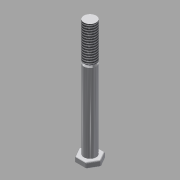
# Autodesk Inventor part: CIM Mount Bolt
Saved by Autodesk Inventor 2013 (Build 170138000, 138)
## iProperties
Created: 2013-01-18
Part Number: CIM Mount Bolt
Material: Aluminum 6061-AHC
Document SubType Name: Modeling
Designer: Naphat
Density: 1 g/cm^3
Author: Naphat
Autodesk Inventor part; units mm, degrees
ref_plane "YZ Plane" through (0, 0, 0) normal (1, 0, 0) x (0, 1, 0)
ref_plane "XZ Plane" through (0, 0, 0) normal (0, 1, 0) x (-1, 0, 0)
ref_plane "XY Plane" through (0, 0, 0) normal (0, 0, 1) x (1, 0, 0)
sketch "Sketch1" plane through (0, 0, 0) normal (0, 1, 0) x (-1, 0, 0)
  circle A0 centre (0, 0) radius 5
  dimension "d0" = 10
  constraints: 1 centre point, 1 coincident
  measures "d0" diameter of A0
extrude "Extrusion1" add sketch "Sketch1" along normal blind 65
sketch "Sketch2" plane through (0, 65, 0) normal (0, 1, 0) x (1, 0, 0)
  circle A0 centre (0, 0) radius 5 projected
  dimension "d38" = 10
  measures "d38" diameter of A0
chamfer "Chamfer1" distance 1 angle 45 1 edges at (5, 65, 0)
extrude "Extrusion2" add sketch "Sketch2" along normal blind 30
chamfer "Chamfer2" distance 1 angle 45 1 edges at (-5, 65, 0)
sketch "Sketch3" plane through (0, 0, 0) normal (0, -1, 0) x (1, 0, 0)
  line L0 (0, 0) -> (0, 0) construction
  line L1 (4.5, -7.7942) -> (-4.5, -7.7942)
  line L2 (-4.5, -7.7942) -> (-9, 0)
  line L3 (-9, 0) -> (-4.5, 7.7942)
  line L4 (-4.5, 7.7942) -> (4.5, 7.7942)
  line L5 (4.5, 7.7942) -> (9, 0)
  line L6 (9, 0) -> (4.5, -7.7942)
  circle A0 centre (0, 0) radius 5 projected
  line L7 (-4.5, -7.7942) -> (4.5, 7.7942) construction
  line L8 (-4.5, 7.7942) -> (4.5, -7.7942) construction
  dimension "d21" = 9
  dimension "d22" = 9
  dimension "d23" = 120
  dimension "d24" = 9
  dimension "d25" = 9
  dimension "d26" = 120
  dimension "d34" = 9
  dimension "d36" = 0
  dimension "d37" = 0
  constraints: 18 end point, 3 parallel, 1 perpendicular
  measures "d21" distance of L1.start L1.end
  measures "d22" distance of L1.end L2.end
  measures "d23" angle of L1 L2
  measures "d24" distance of L2.end L3.end
  measures "d25" distance of L4.end L5.end
  measures "d26" angle of L4 L5
  measures "d34" distance of L3.end L4.end
  measures "d36" distance from line of A0.centre L7
  measures "d37" distance from line of A0.centre L8
extrude "Extrusion3" add sketch "Sketch3" along normal blind 5 contours L1 L2 L3 L4 L5 L6 | A0
chamfer "Chamfer3" distance 1 angle 45 6 edges at (0, -5, -7.7942) (-6.75, -5, -3.8971) (-6.75, -5, 3.8971) (0, -5, 7.7942) (6.75, -5, 3.8971) (6.75, -5, -3.8971)
fillet "Fillet1" radius 1 12 edges at (-4.2113, -4.5, -7.2942) (4.2113, -4.5, -7.2942) (8.4226, -4.5, 0) (4.2113, -4.5, 7.2942) (-4.2113, -4.5, 7.2942) (-8.4226, -4.5, 0) (-5.884, -5, -3.3971) (-5.884, -5, 3.3971) (0, -5, 6.7942) (5.884, -5, 3.3971) (5.884, -5, -3.3971) (0, -5, -6.7942)
fillet "Fillet2" radius 1 12 edges at (4.5, -1.9543, -7.7942) (9, -1.9543, 0) (4.5, -1.9543, 7.7942) (-4.5, -1.9543, 7.7942) (-9, -1.9543, 0) (-4.5, -1.9543, -7.7942) (-6.75, 0, 3.8971) (-6.75, 0, -3.8971) (0, 0, 7.7942) (6.75, 0, 3.8971) (6.75, 0, -3.8971) (0, 0, -7.7942)
thread "Thread3" size "7/16-14 UNC" class "2A" standard "ANSI Unified Screw Threads" full length
equation "\"d21\" = d24"
equation "\"d22\" = d24"
equation "\"d25\" = d24"
body "Solid1"
